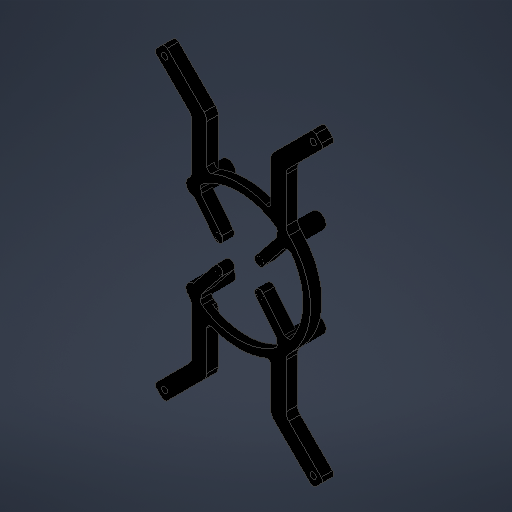
# Autodesk Inventor part: Center Hub old
Saved by Autodesk Inventor 2026.1 (Build 301233020, 233B)
## iProperties
Created: 2025-11-27
Part Number: Center Hub old
Material: Generic
Document SubType Name: Modeling
Designer: Bahaa
Density: 1 g/cm^3
Appearance: Default
Author: Bahaa
Autodesk Inventor part; units mm, degrees
ref_plane "YZ Plane" through (0, 0, 0) normal (1, 0, 0) x (0, 1, 0)
ref_plane "XZ Plane" through (0, 0, 0) normal (0, 1, 0) x (-1, 0, 0)
ref_plane "XY Plane" through (0, 0, 0) normal (0, 0, 1) x (1, 0, 0)
sketch "Sketch1" plane through (0, 0, 0) normal (0, 1, 0) x (-1, 0, 0)
  circle A0 centre (38.890879, 75.660426) radius 1.6
  line L0 (0, 0) -> (50, 0) construction
  line L1 (0, 0) -> (0, -50) construction
  circle A1 centre (38.890879, -75.660426) radius 1.6
  circle A2 centre (-38.890879, 75.660426) radius 1.6
  circle A3 centre (-38.890879, -75.660426) radius 1.6
  line L2 (33.234025, 75.660426) -> (38.890879, 81.31728)
  line L3 (38.890879, 81.31728) -> (44.547734, 75.660426)
  line L4 (44.547734, 75.660426) -> (38.890879, 70.003571)
  line L5 (38.890879, 70.003571) -> (33.234025, 75.660426)
  line L6 (33.234025, 75.660426) -> (44.547734, 75.660426) construction
  line L7 (38.890879, 81.31728) -> (38.890879, 70.003571) construction
  line L8 (33.234025, 75.660426) -> (41.234025, 75.660426) construction
  circle A4 centre (0, 0) radius 37.5
  line L9 (38.890879, 70.003571) -> (24.748744, 55.861436)
  line L10 (24.748744, 55.861436) -> (24.748744, 28.173564)
  line L11 (33.234025, 75.660426) -> (16.748744, 59.175144)
  line L12 (16.748744, 59.175144) -> (16.748744, 33.551894)
  circle A5 centre (0, 0) radius 33.5
  line L13 (0, 0) -> (23.688077, 23.688077) construction
  circle A6 centre (23.688077, 23.688077) radius 4
  circle A7 centre (38.890879, -75.660426) radius 1.6
  line L14 (33.234025, -75.660426) -> (38.890879, -81.31728)
  line L15 (38.890879, -81.31728) -> (44.547734, -75.660426)
  line L16 (44.547734, -75.660426) -> (38.890879, -70.003571)
  line L17 (38.890879, -70.003571) -> (33.234025, -75.660426)
  line L18 (33.234025, -75.660426) -> (44.547734, -75.660426) construction
  line L19 (38.890879, -81.31728) -> (38.890879, -70.003571) construction
  line L20 (33.234025, -75.660426) -> (41.234025, -75.660426) construction
  line L21 (38.890879, -70.003571) -> (24.748744, -55.861436)
  line L22 (24.748744, -55.861436) -> (24.748744, -28.173564)
  line L23 (33.234025, -75.660426) -> (16.748744, -59.175144)
  line L24 (16.748744, -59.175144) -> (16.748744, -33.551894)
  circle A8 centre (23.688077, -23.688077) radius 4
  circle A9 centre (-38.890879, 75.660426) radius 1.6
  circle A10 centre (-38.890879, -75.660426) radius 1.6
  line L25 (-33.234025, 75.660426) -> (-38.890879, 81.31728)
  line L26 (-38.890879, 81.31728) -> (-44.547734, 75.660426)
  line L27 (-44.547734, 75.660426) -> (-38.890879, 70.003571)
  line L28 (-38.890879, 70.003571) -> (-33.234025, 75.660426)
  line L29 (-33.234025, 75.660426) -> (-44.547734, 75.660426) construction
  line L30 (-38.890879, 81.31728) -> (-38.890879, 70.003571) construction
  line L31 (-33.234025, 75.660426) -> (-41.234025, 75.660426) construction
  line L32 (-38.890879, 70.003571) -> (-24.748744, 55.861436)
  line L33 (-24.748744, 55.861436) -> (-24.748744, 28.173564)
  line L34 (-33.234025, 75.660426) -> (-16.748744, 59.175144)
  line L35 (-16.748744, 59.175144) -> (-16.748744, 33.551894)
  circle A11 centre (-23.688077, 23.688077) radius 4
  line L36 (-33.234025, -75.660426) -> (-44.547734, -75.660426) construction
  line L37 (-33.234025, -75.660426) -> (-38.890879, -81.31728)
  line L38 (-38.890879, -81.31728) -> (-44.547734, -75.660426)
  line L39 (-33.234025, -75.660426) -> (-41.234025, -75.660426) construction
  circle A12 centre (-23.688077, -23.688077) radius 4
  circle A13 centre (-38.890879, -75.660426) radius 1.6
  line L40 (-44.547734, -75.660426) -> (-38.890879, -70.003571)
  line L41 (-38.890879, -70.003571) -> (-33.234025, -75.660426)
  line L42 (-38.890879, -81.31728) -> (-38.890879, -70.003571) construction
  line L43 (-38.890879, -70.003571) -> (-24.748744, -55.861436)
  line L44 (-33.234025, -75.660426) -> (-16.748744, -59.175144)
  line L45 (-16.748744, -59.175144) -> (-16.748744, -33.551894)
  line L46 (-24.748744, -55.861436) -> (-24.748744, -28.173564)
  line L47 (-16.748744, 33.551894) -> (-16.748744, 29.012576)
  line L48 (16.748744, 33.551894) -> (16.748744, 29.012576)
  line L49 (-16.748744, -33.551894) -> (-16.748744, -29.012576)
  line L50 (16.748744, -33.551894) -> (16.748744, -29.012576)
  line L51 (-13, 10.25) -> (13, 10.25) construction
  line L52 (13, 10.25) -> (13, -10.25) construction
  line L53 (13, -10.25) -> (-13, -10.25) construction
  line L54 (-13, -10.25) -> (-13, 10.25) construction
  line L55 (-13, 10.25) -> (13, -10.25) construction
  line L56 (13, 10.25) -> (-13, -10.25) construction
  line L57 (13, 10.25) -> (10.795, 10.25) construction
  line L58 (10.795, 10.25) -> (10.795, 7.62) construction
  line L59 (10.795, 7.62) -> (13, 7.62) construction
  line L60 (13, 7.62) -> (13, 10.25) construction
  line L61 (23.688077, 23.688077) -> (10.795, 7.62) construction
  line L62 (21.738193, 25.25267) -> (8.845116, 9.184593)
  line L63 (12.744884, 6.055407) -> (25.637961, 22.123484)
  arc A14 (25.637961, 22.123484) -> (21.738193, 25.25267) centre (23.688077, 23.688077) ccw
  arc A15 (8.845116, 9.184593) -> (12.744884, 6.055407) centre (10.795, 7.62) ccw
  line L64 (21.738193, -25.25267) -> (8.845116, -9.184593)
  line L65 (12.744884, -6.055407) -> (25.637961, -22.123484)
  arc A16 (21.738193, -25.25267) -> (25.637961, -22.123484) centre (23.688077, -23.688077) ccw
  arc A17 (12.744884, -6.055407) -> (8.845116, -9.184593) centre (10.795, -7.62) ccw
  line L66 (-21.738193, 25.25267) -> (-8.845116, 9.184593)
  line L67 (-12.744884, 6.055407) -> (-25.637961, 22.123484)
  arc A18 (-21.738193, 25.25267) -> (-25.637961, 22.123484) centre (-23.688077, 23.688077) ccw
  arc A19 (-12.744884, 6.055407) -> (-8.845116, 9.184593) centre (-10.795, 7.62) ccw
  arc A20 (-25.637961, -22.123484) -> (-21.738193, -25.25267) centre (-23.688077, -23.688077) ccw
  line L68 (-12.744884, -6.055407) -> (-25.637961, -22.123484)
  line L69 (-21.738193, -25.25267) -> (-8.845116, -9.184593)
  arc A21 (-8.845116, -9.184593) -> (-12.744884, -6.055407) centre (-10.795, -7.62) ccw
  line L70 (-13.335, 10.16) -> (13.335, 10.16)
  line L71 (13.335, 10.16) -> (13.335, -10.16)
  line L72 (13.335, -10.16) -> (-13.335, -10.16)
  line L73 (-13.335, -10.16) -> (-13.335, 10.16)
  line L74 (-13.335, 10.16) -> (13.335, -10.16) construction
  line L75 (13.335, 10.16) -> (-13.335, -10.16) construction
  point P0 (-50, 0)
  point P1 (-50, 0)
  point P2 (-26.342598, -20.695834)
  point P3 (-26.342598, 20.695834)
  point P4 (-20.695834, 26.342598)
  point P5 (20.695834, 26.342598)
  point P6 (26.342598, 20.695834)
  point P7 (26.342598, -20.695834)
  point P8 (20.695834, -26.342598)
  point P9 (-20.695834, -26.342598)
  point P10 (-24.748744, 28.173564)
  point P11 (-24.748744, -28.173564)
  point P12 (-16.748744, -33.551894)
  point P13 (16.748744, -33.551894)
  point P14 (-16.748744, 33.551894)
  point P15 (26.516504, -26.516504)
  point P16 (-26.516504, -26.516504)
  point P17 (-26.516504, 26.516504)
  point P18 (26.516504, 26.516504)
  point P19 (17.241539, 15.654039)
  point P20 (19.784017, -22.817266)
  point P21 (23.683785, -19.688079)
  point P22 (-23.683785, -19.688079)
  point P23 (-19.784017, -22.817266)
  point P24 (-19.784017, 22.817266)
  point P25 (-23.683785, 19.688079)
  point P26 (23.683785, 19.688079)
  point P27 (19.784017, 22.817266)
  dimension "d0" = 3.2
  dimension "d4" = 75.66043
  dimension "d5" = 38.89088
  dimension "d6" = 50
  dimension "d7" = 50
  dimension "d8" = 8
  dimension "d9" = 45
  dimension "d10" = 8
  dimension "d11" = 75
  dimension "d12" = 20
  dimension "d13" = 8
  dimension "d16" = 8
  dimension "d17" = 4
  dimension "d18" = 8
  dimension "d19" = 135
  dimension "d20" = 8
  dimension "d45" = 26
  dimension "d46" = 20.5
  dimension "d49" = 5
  dimension "d57" = 26.67
  dimension "d58" = 20.32
  dimension "d59" = 2.54
  dimension "d60" = 2.63
  constraints: 154 end point, 63 symmetric about line, 23 point on circle, 22 centre point, 13 midpoint, 10 parallel, 5 coincident, 5 horizontal, 5 perpendicular, 4 tangent, 4 vertical, 2 point on line, 1 equal length, 16 other
  measures "d0" diameter of A0
  measures "d4" vertical distance of L0.start A0.centre
  measures "d5" horizontal distance of L0.start A0.centre
  measures "d6" distance of L0.start L0.end
  measures "d7" distance of L0.start L1.end
  measures "d8" distance of L2.start L2.end
  measures "d9" angle of L8 L2
  measures "d10" distance of L2.end L3.end
  measures "d11" diameter of A4
  measures "d12" distance of L4.end L9.end
  measures "d13" distance between parallel lines of L9 L11
  measures "d16" distance from line of L11.start L3
  measures "d17" radial gap between concentric circles of A4 A5
  measures "d18" distance between parallel lines of L10 L12
  measures "d19" angle of L1 L13
  measures "d20" diameter of A6
  measures "d45" distance of L52.end L53.end
  measures "d46" distance of L51.end L52.end
  measures "d49" diameter of A15
  measures "d57" distance of L71.end L72.end
  measures "d58" distance of L70.end L71.end
  measures "d59" distance between parallel lines of L71 L58
  measures "d60" distance between parallel lines of L51 L59
extrude "Extrusion1" add sketch "Sketch1" against normal blind 6 contours A0 | A1 | A2 | A3 | L2 L3 L4 L5 | L5 L9 L10 A4 L12 L11 | L48 A5 L47 A4 | A4 A6 A5 L48 | L47 A5 A11 A4 | A4 L33 L32 L28 L34 L35 | A6 A5 L63 A14 | A5 A14 L62 A6 | A11 A5 A12 A4 | A11 A5 A18 L67 | L28 L27 L26 L25 | A11 L66 A18 A5 | A14 L63 A5 | A5 L63 A6 L62 A14 | A6 L63 L71 L70 L62 | A4 L50 A5 A8 | A8 A5 A16 L65 | A6 L63 A5 | A12 A5 L49 A4 | A12 A5 L68 A20 | A5 L67 A11 | A18 L66 A11 L67 A5 | A5 L67 A18 | L70 L71 L63 A15 L62 | L22 L21 L17 L23 L24 A4 | A8 L64 A16 A5 | A4 L45 L44 L41 L43 L46 | A12 L68 A5 | A5 A20 L69 A12 | A11 L66 L70 L73 L67 | L66 A19 L67 L73 L70 | A4 L49 A5 L50 | A16 L64 A8 L65 A5 | A5 L65 A16 | L64 L72 L71 L65 A8 | A5 L65 A8 | L68 A12 L69 A20 A5 | A5 A20 L68 | L68 L73 L72 L69 A12 | L71 L72 L64 A17 L65 | L16 L15 L14 L17 | L41 L37 L38 L40 | L68 A21 L69 L72 L73
hole "Hole1" at (-38.890879, 0, 75.660426) at (38.890879, 0, 75.660426) at (38.890879, 0, -75.660426) at (-38.890879, 0, -75.660426) direction (0, -1, 0) diameter 3.2 end through all counterbore diameter 5.7 counterbore depth 3
extrude "Extrusion3" add sketch "Sketch1" along normal blind 12 contours A6 A5 L63 A14 | A5 A14 L62 A6 | A11 A5 A18 L67 | A11 L66 A18 A5 | A14 L63 A5 | A5 L63 A6 L62 A14 | A8 A5 A16 L65 | A6 L63 A5 | A12 A5 L68 A20 | A5 L67 A11 | A18 L66 A11 L67 A5 | A5 L67 A18 | A8 L64 A16 A5 | A12 L68 A5 | A5 A20 L69 A12 | A16 L64 A8 L65 A5 | A5 L65 A16 | A5 L65 A8 | L68 A12 L69 A20 A5 | A5 A20 L68
sketch "Sketch2" plane through (-23.688077, 12, 23.688077) normal (0, 1, 0) x (1, 0, 0)
  circle A0 centre (0, 0) radius 4
  circle A1 centre (0, 47.376154) radius 4
  circle A2 centre (47.376154, 47.376154) radius 4
  circle A3 centre (47.376154, 0) radius 4
  point P0 (23.688077, 23.688077)
hole "Hole2" at (-23.688077, 12, 23.688077) at (-23.688077, 12, -23.688077) at (23.688077, 12, -23.688077) at (23.688077, 12, 23.688077) direction (0, -1, 0) diameter 4.2 depth 6
extrude "Extrusion4" cut sketch "Sketch1" against normal blind 2 contours L48 A5 L47 A4 | A4 L49 A5 L50
fillet "Fillet1" radius 2 22 edges at (-38.8909, -3, 81.3173) (-44.5477, -3, 75.6604) (-38.8909, -3, -81.3173) (-44.5477, -3, -75.6604) (38.8909, -3, -81.3173) (44.5477, -3, -75.6604) (44.5477, -3, 75.6604) (38.8909, -3, 81.3173) (26.3426, -3, 20.6958) (20.6958, -3, 26.3426) (20.6958, -3, -26.3426) (26.3426, -3, -20.6958) (-20.6958, -3, -26.3426) (-20.6958, -3, 26.3426) (-16.7487, -4, 33.5519) (16.7487, -4, 33.5519) (16.7487, -4, -33.5519) (-16.7487, -4, -33.5519) (16.7487, -1, -29.0126) (-16.7487, -1, -29.0126) (16.7487, -1, 29.0126) (-16.7487, -1, 29.0126)
fillet "Fillet2" radius 5 12 edges at (-16.7487, -3, 59.1751) (-24.7487, -3, 55.8614) (16.7487, -3, 59.1751) (24.7487, -3, 55.8614) (16.7487, -3, -59.1751) (24.7487, -3, -55.8614) (-16.7487, -3, -59.1751) (-24.7487, -3, -55.8614) (-24.7487, -3, -28.1736) (-24.7487, -3, 28.1736) (24.7487, -3, 28.1736) (24.7487, -3, -28.1736)
hole "Hole3" at (-10.795, 0, 7.62) at (-10.795, 0, -7.62) at (10.795, 0, 7.62) at (10.795, 0, -7.62) direction (0, -1, 0) diameter 3.9 depth 5.7
body "Solid1"
